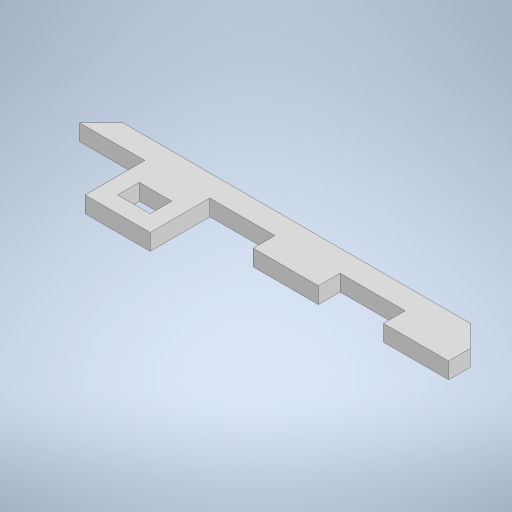
# Autodesk Inventor part: креп
Saved by Autodesk Inventor 2023.1 (Build 271208000, 208)
## iProperties
Created: 2025-01-21
Part Number: креп
Material: Типовые
Document SubType Name: Modeling
Designer: DELL
Density: 1 g/cm^3
Appearance: По умолчанию
Author: DELL
Autodesk Inventor part; units mm, degrees
ref_plane "YZ Plane" through (0, 0, 0) normal (1, 0, 0) x (0, 1, 0)
ref_plane "XZ Plane" through (0, 0, 0) normal (0, 1, 0) x (-1, 0, 0)
ref_plane "XY Plane" through (0, 0, 0) normal (0, 0, 1) x (1, 0, 0)
sketch "Эскиз1" plane through (0, 0, 0) normal (0, 1, 0) x (-1, 0, 0)
  line L0 (-4, -4) -> (-68, -4)
  line L1 (-72, 0) -> (-72, 4)
  line L2 (0, 0) -> (-3.643, -3.643)
  line L3 (-3.643, -3.643) -> (-4, -4)
  line L4 (-48, 4) -> (-48, 0)
  line L5 (-48, 4) -> (-48, 0)
  line L6 (-36, 4) -> (-36, 0)
  line L7 (-60, 4) -> (-60, 0)
  line L8 (-72, 4) -> (-60, 4)
  line L9 (-48, 4) -> (-36, 4)
  line L10 (-60, 0) -> (-48, 0)
  line L11 (-36, 0) -> (-24, 0)
  line L12 (-12, 0) -> (0, 0)
  line L13 (-68, -4) -> (-72, 0)
  line L14 (-24, 11) -> (-12, 11)
  line L15 (-12, 11) -> (-12, 0)
  line L16 (-24, 11) -> (-24, 0)
  point P0 (0, 0)
  point P1 (-48, 2)
  point P2 (-72, 2)
  point P3 (-48, 2)
  point P4 (-12, 2)
  point P5 (-36, 2)
  point P6 (-60, 2)
  point P7 (-30, 0)
  point P8 (-3.8215, -3.8215)
  dimension "d9" = 24
  dimension "d13" = 12
  dimension "d19" = 4
  dimension "d23" = 8
  dimension "d26" = 135
  dimension "d28" = 72
  dimension "d29" = 12
  dimension "d30" = 11
  constraints: 34 end point, 7 midpoint, 6 equal length, 5 parallel, 5 vertical, 2 horizontal, 2 point on line, 1 coincident
  measures "d9" distance of point (-72, 2) point (-48, 2)
  measures "d13" distance of point (-60, 2) point (-48, 2)
  measures "d19" distance between parallel lines of L11 L0
  measures "d23" distance between parallel lines of L8 L0
  measures "d26" angle of L1 L13
  measures "d28" distance of L1.start point (0, 0)
  measures "d29" distance of L14.start L14.end
  measures "d30" distance of L14.end L12.start
extrude "Выдавливание1" add sketch "Эскиз1" along normal blind 3
sketch "Эскиз2" plane through (0, 3, 0) normal (0, 1, 0) x (1, 0, 0)
  line L0 (12, 0) -> (12, -11) construction
  line L1 (12, -11) -> (24, -11) construction
  line L2 (15, -4) -> (15, -8)
  line L3 (15, -8) -> (21, -8)
  line L4 (15, -4) -> (21, -4)
  line L5 (21, -4) -> (21, -8)
  line L6 (24, -11) -> (24, 0) projected
  point P0 (0, 0)
  point P1 (21, -6)
  dimension "d31" = 3
  dimension "d32" = 4
  dimension "d33" = 3
  dimension "d36" = 3
  constraints: 8 end point, 1 horizontal, 1 midpoint, 1 perpendicular
  measures "d31" distance between parallel lines of L0 L2
  measures "d32" distance of L4.end L3.end
  measures "d33" distance from line of L6 point (21, -6)
  measures "d36" distance between parallel lines of L1 L3
extrude "Выдавливание2" cut sketch "Эскиз2" against normal blind 10
